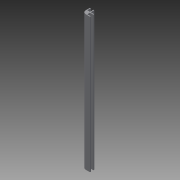
# Autodesk Inventor part: profile
Saved by Autodesk Inventor 2013 SP1 (Build 170176100, 176)
## iProperties
Created: 2019-01-15
Part Number: profile
Material: Типовые
Document SubType Name: Modeling
Designer: jhcjhguw
Density: 1 g/cm^3
Author: jhcjhguw
Autodesk Inventor part; units mm, degrees
ref_plane "YZ Plane" through (0, 0, 0) normal (1, 0, 0) x (0, 1, 0)
ref_plane "XZ Plane" through (0, 0, 0) normal (0, 1, 0) x (-1, 0, 0)
ref_plane "XY Plane" through (0, 0, 0) normal (0, 0, 1) x (1, 0, 0)
sketch "Эскиз1" plane through (0, 0, 0) normal (0, 0, 1) x (1, 0, 0)
  line L0 (0, 2.65) -> (0, 6)
  line L1 (2.65, 0) -> (6, 0)
  line L2 (0, 6) -> (0.65, 6)
  line L3 (0.65, 6) -> (0.65, 3.3)
  line L4 (0.65, 3.3) -> (2.65, 3.3)
  line L5 (2.65, 3.3) -> (2.65, 6)
  line L6 (2.65, 6) -> (3.3, 6)
  line L7 (3.3, 6) -> (3.3, 3.3)
  line L8 (3.3, 3.3) -> (6, 3.3)
  line L9 (6, 3.3) -> (6, 2.65)
  line L10 (6, 2.65) -> (3.3, 2.65)
  line L11 (3.3, 2.65) -> (3.3, 0.65)
  line L12 (3.3, 0.65) -> (6, 0.65)
  line L13 (6, 0.65) -> (6, 0)
  arc A0 (0, 2.65) -> (2.65, 0) centre (2.65, 2.65) ccw
  point P0 (0, 0)
  dimension "d0" = 6
  dimension "d1" = 6
  dimension "d2" = 0.65
  dimension "d3" = 2.7
  dimension "d4" = 2
  dimension "d5" = 0.65
  dimension "d6" = 2.7
  dimension "d7" = 0.65
  dimension "d8" = 2
  dimension "d9" = 0.65
  dimension "d12" = 2.65
  dimension "d13" = 2.65
  dimension "d14" = 2.65
  constraints: 28 end point, 9 parallel, 3 collinear, 3 perpendicular, 2 point on circle, 2 tangent, 1 centre point, 1 vertical
  measures "d0" distance of point (0, 0) L0.end
  measures "d1" distance of point (0, 0) L1.end
  measures "d2" distance of L0.end L2.end
  measures "d3" distance of L2.end L3.end
  measures "d4" distance of L3.end L4.end
  measures "d5" distance of L5.end L6.end
  measures "d6" distance of L7.end L8.end
  measures "d7" distance of L8.end L9.end
  measures "d8" distance of L10.end L11.end
  measures "d9" distance of L12.end L1.end
  measures "d12" radius of A0
  measures "d13" horizontal distance of point (0, 0) A0.centre
  measures "d14" horizontal distance of point (0, 0) A0.centre
extrude "Выдавливание1" add sketch "Эскиз1" along normal blind 104.8
